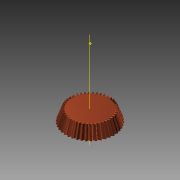
# Autodesk Inventor part: Bevel Gear1
Saved by Autodesk Inventor 2015 (Build 190141000, 141)
## iProperties
Created: 2008-07-23
Part Number: Bevel Gear1
Material: Steel, Mild
Document SubType Name: Modeling
Designer: tangg
Categories: <?xml version="1.0" encoding="UTF-16"?> <MemberInstance><Categories><FamilyTemplate><FamilyTemplateParameter ValueType="xs:double" Id="1" ObjectReferenceKey="da_z" ObjectType="kUserParameterObject"/><FamilyTemplateParameter ValueType="xs:double" Id="2" ObjectReferenceKey="da_b" ObjectType="kUserParameterObject"/><FamilyTemplateParameter ValueType="xs:double" Id="3" ObjectReferenceKey="da_beta" ObjectType="kUserParameterObject"/><FamilyTemplateParameter ValueType="xs:double" Id="4" ObjectReferenceKey="da_dae" ObjectType="kUserParameterObject"/><FamilyTemplateParameter ValueType="xs:double" Id="5" ObjectReferenceKey="da_ve" ObjectType="kUserParameterObject"/><FamilyTemplateParameter ValueType="xs:double" Id="6" ObjectReferenceKey="da_omega" ObjectType="kUserParameterObject"/><FamilyTemplateParameter ValueType="xs:string" Id="7" ObjectReferenceKey="EAIAABAAAAAAHwAAAAAAAIAAAAAAAAAA" ObjectType="83914240" SubObjectId="SurfaceGeometry"/></FamilyTemplate><ParamToTemplateMap><ParamToTemplate CategoryParameter="//CategoryParameter[@InternalName='046C89C9-8512-4d59-83FE-43B91F4F132A']" TemplateParameter="1"/><ParamToTemplate CategoryParameter="//CategoryParameter[@InternalName='2552DF32-E462-4b46-AEBF-C6C7768E72AC']" TemplateParameter="2"/><ParamToTemplate CategoryParameter="//CategoryParameter[@InternalName='C9EE641D-15FC-4fae-A226-E94C4372FDD7']" TemplateParameter="3"/><ParamToTemplate><ParamToTemplate CategoryParameter="//CategoryParameter[@InternalName='00B6519A-459B-49c7-AD84-2E56D39A5744']" ConstantValue="0.000000"/></ParamToTemplate><ParamToTemplate><ParamToTemplate CategoryParameter="//CategoryParameter[@InternalName='04B31F0E-C7A6-4894-AA32-9629BEFACF47']" ConstantValue="1.000000"/></ParamToTemplate><ParamToTemplate><ParamToTemplate CategoryParameter="//CategoryParameter[@InternalName='43CBEC2E-7847-49e7-A936-2F7889FCB2D9']" ConstantValue="0.200000"/></ParamToTemplate><ParamToTemplate><ParamToTemplate CategoryParameter="//CategoryParameter[@InternalName='B1EFC894-105D-4ebd-86BF-FA20ED196853']" ConstantValue="0.300000"/></ParamToTemplate><ParamToTemplate><ParamToTemplate CategoryParameter="//CategoryParameter[@InternalName='51175063-3D10-4879-93E8-6246FE8B403D']" ConstantValue="2060000000.000000"/></ParamToTemplate><ParamToTemplate><ParamToTemplate CategoryParameter="//CategoryParameter[@InternalName='A3A52E27-4454-46a9-B0BD-C932399B70AF']" ConstantValue="0.300000"/></ParamToTemplate><ParamToTemplate CategoryParameter="//CategoryParameter[@InternalName='2A200944-5A8C-41ca-B96E-8520D2E510F1']" TemplateParameter="4"/><ParamToTemplate><ParamToTemplate CategoryParameter="//CategoryParameter[@InternalName='1A637F62-92C8-44bc-B81F-10802510B579']" ConstantValue="2.530585"/></ParamToTemplate><ParamToTemplate CategoryParameter="//CategoryParameter[@InternalName='B52DD4BE-6863-48fb-BF58-89EF6F9EC65C']" TemplateParameter="5"/><ParamToTemplate><ParamToTemplate CategoryParameter="//CategoryParameter[@InternalName='3956BFF2-84D2-457d-93C2-9B0613DEBA67']" ConstantValue="3.515844"/></ParamToTemplate><ParamToTemplate CategoryParameter="//CategoryParameter[@InternalName='739CFA02-461B-4bf8-8049-181FCAD8B28F']" TemplateParameter="6"/><ParamToTemplate><ParamToTemplate CategoryParameter="//CategoryParameter[@InternalName='A27E999F-E2CE-4481-8A2A-EBF499C4C3C5']" ConstantValue="0.000000"/></ParamToTemplate><ParamToTemplate><ParamToTemplate CategoryParameter="//CategoryParameter[@InternalName='9E1B4470-B2D3-4ff1-B813-535BB4CDF51A']" ConstantValue="3520000.000000"/></ParamToTemplate><ParamToTemplate><ParamToTemplate CategoryParameter="//CategoryParameter[@InternalName='F8452263-BFF6-458c-9FB1-07C4B99E95CD']" ConstantValue="11400000.000000"/></ParamToTemplate><ParamToTemplate><ParamToTemplate CategoryParameter="//CategoryParameter[@InternalName='3E3BB259-FD49-497f-8171-6EBC954A3479']" ConstantValue="2.000000"/></ParamToTemplate><ParamToTemplate CategoryParameter="//CategoryParameter[@InternalName='27C3BAF2-7550-4e4b-AE2C-0DB134B7D9B7']" TemplateParameter="7"/></ParamToTemplateMap><Category DisplayName="Gear" InternalName="DC85795E-93AB-48d5-8EEE-5A27447B64BD" Mnemonic="Gear"><CategoryParameter DisplayName="z" InternalName="046C89C9-8512-4d59-83FE-43B91F4F132A" Mnemonic="z"/><CategoryParameter DisplayName="b" InternalName="2552DF32-E462-4b46-AEBF-C6C7768E72AC" Mnemonic="b"/><CategoryParameter DisplayName="||b|" InternalName="C9EE641D-15FC-4fae-A226-E94C4372FDD7" Mnemonic="beta"/><CategoryParameter DisplayName="x" InternalName="00B6519A-459B-49c7-AD84-2E56D39A5744" Mnemonic="x"/><CategoryParameter DisplayName="a*" InternalName="04B31F0E-C7A6-4894-AA32-9629BEFACF47" Mnemonic="a"/><CategoryParameter DisplayName="c*" InternalName="43CBEC2E-7847-49e7-A936-2F7889FCB2D9" Mnemonic="c"/><CategoryParameter DisplayName="r|.f|*" InternalName="B1EFC894-105D-4ebd-86BF-FA20ED196853" Mnemonic="rf"/><CategoryParameter DisplayName="E" InternalName="51175063-3D10-4879-93E8-6246FE8B403D" Mnemonic="E"/><CategoryParameter DisplayName="||m|" InternalName="A3A52E27-4454-46a9-B0BD-C932399B70AF" Mnemonic="mi"/><Category DisplayName="BevelGear" InternalName="0C98F69A-0C2B-4791-B2FE-7691BB227E77" Mnemonic="BevelGear"><CategoryParameter DisplayName="d|.ae|" InternalName="2A200944-5A8C-41ca-B96E-8520D2E510F1" Mnemonic="dae"/><CategoryParameter DisplayName="d|.ai|" InternalName="1A637F62-92C8-44bc-B81F-10802510B579" Mnemonic="dai"/><CategoryParameter DisplayName="A|.e|" InternalName="B52DD4BE-6863-48fb-BF58-89EF6F9EC65C" Mnemonic="ve"/><CategoryParameter DisplayName="A|.i|" InternalName="3956BFF2-84D2-457d-93C2-9B0613DEBA67" Mnemonic="vi"/><CategoryParameter DisplayName="||S|" InternalName="739CFA02-461B-4bf8-8049-181FCAD8B28F" Mnemonic="omega"/><CategoryParameter DisplayName="x|.t|" InternalName="A27E999F-E2CE-4481-8A2A-EBF499C4C3C5" Mnemonic="xt"/><CategoryParameter DisplayName="||s||.Flim|" InternalName="9E1B4470-B2D3-4ff1-B813-535BB4CDF51A" Mnemonic="sFlim"/><CategoryParameter DisplayName="||s||.Hlim|" InternalName="F8452263-BFF6-458c-9FB1-07C4B99E95CD" Mnemonic="sHlim"/><CategoryParameter DisplayName="type" InternalName="3E3BB259-FD49-497f-8171-6EBC954A3479" Mnemonic="type"/><CategoryParameter DisplayName="PitchDiameter" InternalName="27C3BAF2-7550-4e4b-AE2C-0DB134B7D9B7" Mnemonic="IDS_PITCHDIAM"/></Category></Category></Categories></MemberInstance>
Mass: 60.9118 g
Surface Area: 34.3074 cm^2
Volume: 7.7496 cm^3
Density: 7.86 g/cm^3
Appearance: Copper - Polished
CustomPartVersion: 1
Author: tangg
Autodesk Inventor part; units mm, degrees
ref_plane "Mesh Plane2" through (0, 0, 0) normal (0.9972038, 0.0747301, 0) x (0, 0, 1)
sketch "Teeth Body Sketch" plane through (0, 0, 0) normal (1, 0, 0) x (0, 1, 0)
  line L0 (0, 0) -> (13.9053, -43.1858) construction
  line L1 (13.9053, -43.1858) -> (15.3622, -42.6867)
  line L2 (15.3622, -42.6867) -> (0, 0) construction
  line L3 (14.7, -42.9136) -> (0, 0) construction
  line L4 (11.453, -35.5695) -> (12.6529, -35.1584)
  line L5 (13.9053, -43.1858) -> (11.453, -35.5695)
  line L6 (15.3622, -42.6867) -> (12.6529, -35.1584)
  line L7 (0, -51.8229) -> (0, 8.6372) projected
  line L8 (0, -42.9136) -> (15.3622, -42.9136) construction
  dimension "d0" = 29.4
  dimension "d1" = 27.8107
  dimension "d2" = 30.7245
  dimension "d3" = 8
  dimension "d4" = 42.6867
  constraints: 16 end point, 4 point on line, 3 perpendicular, 2 collinear, 1 horizontal alignment, 1 vertical alignment
  measures "d0" diameter of L3.start L7
  measures "d1" diameter of L0.end L7
  measures "d2" diameter of L1.end L7
  measures "d3" distance between parallel lines of L1 L4
  measures "d4" vertical distance of L1.end L0.start
revolve "Teeth Body" add sketch "Teeth Body Sketch" angle 360 about axis through (0, 0, 0) along (0, 0, 1)
ref_plane "Tooth Plane" through (0, 13.9053, -43.1858) normal (0, 0.3240635, -0.9460353) x (-1, 0, 0)
sketch "Start Sketch" plane through (0, 13.9053, -43.1858) normal (0, 0.3240635, -0.9460353) x (-1, 0, 0)
  line L0 (0, -35.9578) -> (0, 11.1245) projected
  arc A0 (-0.2169, -0.1848) -> (-1.189, 1.9596) centre (-6.0379, -1.5311) ccw
  arc A1 (1.189, 1.9596) -> (0.2169, -0.1848) centre (6.0379, -1.5311) ccw
  line L1 (-0.2169, -0.1848) -> (0.2169, -0.1848)
  arc A2 (1.189, 1.9596) -> (-1.189, 1.9596) centre (0, -14.6985) ccw
  dimension "d7" = 5.9747
  dimension "d8" = 6.0379
  dimension "d9" = 13.1674
  dimension "d57" = 16.7005
  dimension "d58" = 14.5137
  constraints: 6 point on circle, 3 centre point, 3 symmetric about line, 2 end point, 1 coincident, 1 perpendicular, 1 other
  measures "d7" radius of A0
  measures "d8" horizontal distance of point (0, -14.699) A0.centre
  measures "d9" vertical distance of point (0, -14.699) A0.centre
  measures "d57" radius of A2
  measures "d58" distance from line of A2.centre L1
sketch "End Sketch" plane through (0, 11.2879, -35.5446) normal (0, 0.3240635, -0.9460353) x (-1, 0, 0)
  line L0 (0, -34.0348) -> (0, 10.392) projected
  arc A0 (-0.1785, 0.0122) -> (-0.9785, 1.7769) centre (-4.9688, -1.0958) ccw
  arc A1 (0.9785, 1.7769) -> (0.1785, 0.0122) centre (4.9688, -1.0958) ccw
  line L1 (-0.1785, 0.0122) -> (0.1785, 0.0122)
  arc A2 (0.9785, 1.7769) -> (-0.9785, 1.7769) centre (0, -11.9318) ccw
  dimension "d12" = 4.9168
  dimension "d15" = 4.9688
  dimension "d16" = 10.836
  dimension "d59" = 13.7436
  dimension "d60" = 11.9439
  constraints: 6 point on circle, 3 centre point, 3 symmetric about line, 2 end point, 1 coincident, 1 other
  measures "d12" radius of A0
  measures "d15" horizontal distance of A0.centre point (0, -11.932)
  measures "d16" vertical distance of A0.centre point (0, -11.932)
  measures "d59" radius of A2
  measures "d60" distance from line of A2.centre L1
loft "Loft" cut profiles "Start Sketch", "End Sketch"
pattern_circular "Circular Pattern" count 42 over 360 about axis through (0, 0, 0) along (0, 0, 1) of "Loft"
ref_plane "End Plane" through (0, 11.2879, -35.5446) normal (0, 0.3240635, -0.9460353) x (-1, 0, 0)
sketch3d "3D Sketch Right"
ref_plane "End Plane Right" through (-2.0177, 11.9129, -35.2724) normal (0.0541157, -0.3195131, 0.9460353) x (0.9859584, 0.1669911, 0)
sketch "End Sketch Right" plane through (-2.0177, 11.9129, -35.2724) normal (0.0541157, -0.3195131, 0.9460353) x (0.9859584, 0.1669911, 0)
  arc A0 (-0.1785, -0.8278) -> (-0.9785, 0.9369) centre (-4.9688, -1.9358) ccw
  line L0 (0, -17.6885) -> (0, 5.8935) projected
  arc A1 (0.9785, 0.9369) -> (0.1785, -0.8278) centre (4.9688, -1.9358) ccw
  line L1 (-0.1785, -0.8278) -> (0.1785, -0.8278)
  arc A2 (0.9785, 0.9369) -> (-0.9785, 0.9369) centre (0, -12.7718) ccw
  dimension "d70" = 4.9688
  dimension "d71" = 10.836
  dimension "d72" = 4.9168
  dimension "d73" = 11.9439
  dimension "d74" = 13.7436
  constraints: 6 point on circle, 3 centre point, 3 symmetric about line, 2 end point, 1 coincident, 1 perpendicular, 1 other
  measures "d70" horizontal distance of A2.centre A0.centre
  measures "d71" vertical distance of point (0, -12.772) A0.centre
  measures "d72" radius of A0
  measures "d73" distance from line of point (0, -12.772) L1
  measures "d74" radius of A2
feature "Loft Right" [suppressed]
pattern_circular "Circular Pattern Right" [suppressed]
sketch3d "3D Sketch Left"
ref_plane "End Plane Left" through (2.0028, 11.9129, -35.2685) normal (-0.0537241, -0.3195517, 0.9460446) x (0.98616, -0.1657966, 0)
sketch "End Sketch Left" plane through (2.0028, 11.9129, -35.2685) normal (-0.0537241, -0.3195517, 0.9460446) x (0.98616, -0.1657966, 0)
  line L0 (0, -33.711) -> (0, 11.326) projected
  arc A0 (-0.1785, -0.8267) -> (-0.9785, 0.938) centre (-4.9688, -1.9347) ccw
  arc A1 (0.9785, 0.938) -> (0.1785, -0.8267) centre (4.9688, -1.9347) ccw
  line L1 (-0.1785, -0.8267) -> (0.1785, -0.8267)
  ellipse E0 centre (0, -11.3926) end of major axis (12.6529, -11.3926) minor radius 11.9702 projected
  arc A2 (0.9785, 0.938) -> (-0.9785, 0.938) centre (0, -12.7707) ccw
  dimension "d56" = 11.9702
  dimension "d30" = 4.9168
  dimension "d31" = 4.9688
  dimension "d32" = 10.836
  dimension "d61" = 13.7436
  dimension "d62" = 11.9439
  constraints: 6 point on circle, 3 centre point, 3 symmetric about line, 2 end point, 1 coincident, 2 other
  measures "d30" radius of A0
  measures "d31" horizontal distance of point (0, -12.771) A0.centre
  measures "d32" vertical distance of A0.centre point (0, -12.771)
  measures "d61" radius of A2
  measures "d62" distance from line of point (0, -12.771) L1
feature "Loft Left" [suppressed]
pattern_circular "Circular Pattern Left" [suppressed]
sketch "Body Sketch" plane through (0, 0, 0) normal (1, 0, 0) x (0, 1, 0)
  line L0 (0, -44.709) -> (0, -34.0462) projected
  line L1 (13.9053, -43.1858) -> (11.453, -35.5695) projected
  line L2 (11.453, -35.5695) -> (0, -35.5695)
  line L3 (13.9053, -43.1858) -> (0, -43.1858)
  constraints: 4 end point, 2 perpendicular, 2 point on line
revolve "Fix Body" add sketch "Body Sketch" angle 360 about axis through (0, 0, 0) along (0, 0, 1)
sketch "Sketch6" plane through (0, 0, 0) normal (1, 0, 0) x (0, 1, 0)
  line L0 (14.7, -42.9136) -> (0, 0) projected
  line L1 (0, -51.4963) -> (0, 8.5827) projected
surface revolve "Pitch Diameter" sketch "Sketch6" angle 360 about axis through (0, 0, 0) along (0, 0, 1) shown no curves L0
equation "\"d0\" = da_de"
equation "\"d1\" = da_dfe"
equation "\"d2\" = da_dae"
equation "\"d3\" = da_b"
equation "\"d4\" = da_ve"
equation "\"d7\" = fd_rr"
equation "\"d8\" = fd_x"
equation "\"d9\" = fd_y"
equation "\"d57\" = 0.5 * fd_dva + 0.3 * da_he"
equation "\"d58\" = 0.5 * fd_dva - 1.12 * da_he"
equation "\"da_teethtype\" = 0"
equation "\"da_b\" = 8"
equation "\"da_de\" = 29.4"
equation "\"da_dae\" = 30.72445"
equation "\"da_dfe\" = 27.81066"
equation "\"da_le\" = 45.36148"
equation "\"da_omega\" = 45deg"
equation "\"da_beta\" = 0"
equation "\"da_delta\" = 18.908848deg"
equation "\"da_alpha\" = 20deg"
equation "\"da_he\" = 1.54"
equation "\"da_ve\" = 42.68672"
equation "\"da_zv\" = 44.395805"
equation "\"fd_loft\" = da_b + 0.05 * da_he"
equation "\"fd_x\" = fd_x1 + fd_x2"
equation "\"fd_y\" = fd_y1 - fd_y2"
equation "\"fd_dd\" = fd_dva - 0.6 * da_he"
equation "\"da_dvw\" = 31.07706"
equation "\"d11\" = -fd_loft"
equation "\"da_dm\" = 26.80749"
equation "\"da_x\" = 0"
equation "\"da_m\" = 0.7"
equation "\"fd_rr\" = 5.97468"
equation "\"fd_dva\" = 32.477064"
equation "\"fd_x1\" = 0.549664"
equation "\"fd_x2\" = 5.488214"
equation "\"fd_y1\" = 15.528807"
equation "\"fd_y2\" = 2.361421"
body "Solid1"
body "Srf1"
